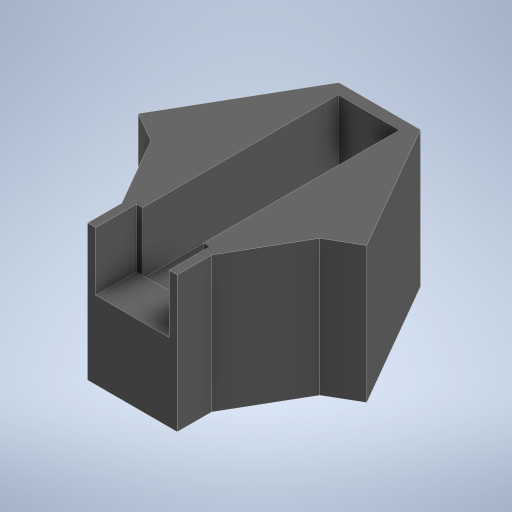
# Autodesk Inventor part: cover
Saved by Autodesk Inventor 2024.1 (Build 281209000, 209)
## iProperties
Created: 2025-01-27
Part Number: cover
Material: 一般
Document SubType Name: Modeling
Designer: hibik
Density: 1 g/cm^3
Appearance: 既定
Author: hibik
Autodesk Inventor part; units mm, degrees
ref_plane "YZ Plane" through (0, 0, 0) normal (1, 0, 0) x (0, 1, 0)
ref_plane "XZ Plane" through (0, 0, 0) normal (0, 1, 0) x (-1, 0, 0)
ref_plane "XY Plane" through (0, 0, 0) normal (0, 0, 1) x (1, 0, 0)
sketch "スケッチ1" plane through (0, 0, 0) normal (0, 1, 0) x (-1, 0, 0)
  line L0 (135, 77.9423) -> (-135, 77.9423)
  line L1 (-135, 77.9423) -> (0, -155.8846)
  line L2 (0, -155.8846) -> (135, 77.9423)
  line L3 (135, 77.9423) -> (-67.5, -38.9711)
  line L4 (75, 77.9423) -> (105, 25.9808)
  line L5 (30, -103.923) -> (-30, -103.923)
  line L6 (-105, 25.9808) -> (-75, 77.9423)
  line L7 (0, 77.9423) -> (0, -155.8846)
  line L8 (-135, 77.9423) -> (67.5, -38.9711)
  line L9 (-33, 77.9423) -> (-33, 52.6884)
  line L10 (-33, 52.6884) -> (-62.1295, 2.2346)
  line L11 (-62.1295, 2.2346) -> (-84, -10.3923)
  line L12 (27, 77.9423) -> (-27, 77.9423)
  line L13 (-27, 77.9423) -> (-27, 47.9423)
  line L14 (-27, 47.9423) -> (27, 47.9423)
  line L15 (27, 47.9423) -> (27, 77.9423)
  point P0 (0, 0)
  point P1 (0, 77.9423)
  point P2 (0, 47.9423)
  dimension "d0" = 270
  dimension "d2" = 30
  dimension "d5" = 42
  dimension "d6" = 49
  dimension "d9" = 54
  dimension "d14" = 30
  constraints: 32 end point, 11 point on line, 5 equal length, 5 perpendicular, 4 midpoint, 3 horizontal, 3 parallel, 2 vertical, 2 vertical alignment
  measures "d0" distance of L0.start L0.end
  measures "d2" distance from line of L4.end L3
  measures "d5" distance of L9.start L6.end
  measures "d6" distance between parallel lines of L10 L6
  measures "d9" distance between parallel lines of L13 L15
  measures "d14" distance of L14.end L12.start
extrude "押し出し1" add sketch "スケッチ1" along normal blind 100 contours L4 L3 L7 L14 L15 L0 | L2 L8 L3 L4 | L15 L14 L7 L0 | L2 L5 L7 L8 | L7 L5 L1 L3 | L8 L10 L9 L0 L13 L14 L7 | L3 L1 L11 L10 L8 | L7 L14 L13 L0 | L10 L11 L1 L6 L8 | L8 L6 L0 L9 L10
extrude "押し出し2" cut sketch "スケッチ1" along normal blind 100 contours L10 L11 L1 L6 L8 | L8 L6 L0 L9 L10
mirror "ミラー1" about plane through (0, 0, 0) normal (1, 0, 0) of "押し出し2"
extrude "押し出し3" cut sketch "スケッチ1" along normal blind 100 contours L15 L14 L7 L0 | L7 L14 L13 L0
extrude "押し出し4" add sketch "スケッチ1" along normal blind 57 contours L15 L14 L7 L0 | L7 L14 L13 L0
sketch "スケッチ2" plane through (0, 100, 0) normal (0, 1, 0) x (1, 0, 0)
  line L0 (-27, -47.9423) -> (27, -47.9423) projected
  line L1 (-22.5, -47.9423) -> (22.5, -47.9423)
  line L2 (22.5, -47.9423) -> (22.5, 95.923)
  line L3 (22.5, 95.923) -> (-22.5, 95.923)
  line L4 (-22.5, 95.923) -> (-22.5, -47.9423)
  line L5 (30, 103.923) -> (-30, 103.923) projected
  point P0 (0, 0)
  point P1 (0, -47.9423)
  dimension "d15" = 45
  dimension "d16" = 8
  constraints: 8 end point, 2 parallel, 1 horizontal, 1 midpoint, 1 perpendicular, 1 point on line, 1 vertical alignment
  measures "d15" distance of L2.end L3.end
  measures "d16" distance between parallel lines of L5 L3
extrude "押し出し5" cut sketch "スケッチ2" against normal blind 45
